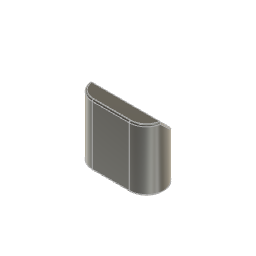
_Pencil Sharpener.d67306bd-12ad-4b4e-934f-6ecedd9aaf55 (Autodesk Fusion 360 design; units mm, degrees)
Autodesk Fusion 360 part; units mm, degrees
sketch "Sketch1" plane through (0, 0, 0) normal (0, 0, 1) x (1, 0, 0)
  circle A0 centre (0, 0) radius 6.985
  line L0 (-15.7585, 8.6989) -> (15.7585, -8.6989) construction
  line L1 (15.7585, 8.6989) -> (-15.7585, -8.6989) construction
  arc A1 (-9.364, 8.6989) -> (-9.364, -8.6989) centre (-9.3009, 0) ccw
  line L2 (0, 0) -> (0, 2.54)
  arc A2 (9.364, -8.6989) -> (9.364, 8.6989) centre (9.3009, 0) ccw
  line L3 (-9.364, -8.6989) -> (9.364, -8.6989)
  line L4 (9.364, 8.6989) -> (-9.364, 8.6989)
  dimension "d1" = 13.97
  constraint coincident A0.centre L2.start
  constraint coincident L0 A0.centre
  constraint coincident L1 A0.centre
  constraint vertical L2
  constraint symmetric A1.start L2 A2.end
  constraint symmetric A1.end L2 A2.start
  constraint symmetric A1 L2 A2
  measures "d1" diameter of A0
extrude "Extrude1" add sketch "Sketch1" along normal blind 38.1
ref_plane "WorkPlane1" through (0, 0, 19.05) normal (-1, 0, 0) x (0, 0, 1)
sketch "Sketch2" plane through (0, 0, 38.1) normal (0, 0, 1) x (-1, 0, 0)
  circle A0 centre (0, 0) radius 6.985
  line L0 (-9.364, -8.6989) -> (9.364, -8.6989)
  arc A1 (9.364, -8.6989) -> (9.364, 8.6989) centre (9.3009, 0) ccw
  line L1 (9.364, 8.6989) -> (-9.364, 8.6989)
  arc A2 (-9.364, 8.6989) -> (-9.364, -8.6989) centre (-9.3009, 0) ccw
sketch "Sketch3" plane through (0, 0, 0) normal (-1, 0, 0) x (0, -1, 0)
  line L0 (-6.985, 38.1) -> (6.985, 38.1)
  line L1 (-6.985, 0) -> (6.985, 0)
  line L2 (-6.985, 38.1) -> (6.985, 38.1)
  line L3 (6.985, 38.1) -> (6.985, 0)
  line L4 (6.985, 0) -> (-6.985, 0)
  line L5 (-6.985, 0) -> (-6.985, 38.1)
  line L6 (6.985, 38.1) -> (-6.985, 24.13)
  line L7 (6.985, 38.1) -> (26.7416, 38.1) construction
  line L8 (-6.985, 24.13) -> (-8.89, 24.13)
  line L9 (-8.89, 24.13) -> (-8.89, 38.1)
  line L10 (-8.89, 38.1) -> (-6.985, 38.1)
  line L11 (-6.985, 38.1) -> (-6.985, 24.13)
  line L12 (-6.985, 24.13) -> (0, 24.13)
  line L13 (0, 24.13) -> (0, 25.4)
  line L14 (0, 25.4) -> (-6.985, 25.4)
  line L15 (-6.985, 25.4) -> (-6.985, 24.13)
  line L16 (-6.985, 24.13) -> (-5.715, 25.4)
  line L17 (0, 25.4) -> (0, 31.115)
  line L18 (0, 31.115) -> (-6.985, 31.115)
  line L19 (6.985, 36.9017) -> (-6.985, 22.9317)
  line L20 (6.985, 36.9017) -> (26.7416, 36.9017) construction
  line L21 (-6.985, 22.9317) -> (-8.8388, 21.0779)
  line L22 (-8.8388, 21.0779) -> (-8.89, 24.13)
  line L23 (0, 31.115) -> (9.144, 31.115)
  line L24 (9.144, 31.115) -> (9.144, 38.354)
  line L25 (9.144, 38.354) -> (0, 38.354)
  line L26 (0, 38.354) -> (0, 31.115)
  dimension "d7" = 135
  dimension "d11" = 135
  constraint horizontal L2
  constraint vertical L3
  constraint horizontal L4
  constraint vertical L5
  constraint coincident L1.end L3.end
  constraint coincident L0.start L2.start
  constraint horizontal L7
  constraint coincident L0.end L2.end
  constraint coincident L5 L6.end
  constraint horizontal L8
  constraint vertical L9
  constraint horizontal L10
  constraint vertical L11
  constraint horizontal L12
  constraint vertical L13
  constraint horizontal L14
  constraint vertical L15
  constraint coincident L6 L16.end
  constraint coincident L14 L16.end
  constraint midpoint L6 L17.end
  constraint perpendicular L14 L17
  constraint midpoint L11 L18.end
  constraint horizontal L20
  constraint coincident L3 L19.start
  constraint coincident L5 L19.end
  constraint parallel L19 L21
  constraint horizontal L23
  constraint vertical L24
  constraint horizontal L25
  constraint vertical L26
  measures "d7" angle of L6 L7
  measures "d11" angle of L19 L20
revolve "Revolve1" add sketch "Sketch3" angle 360 about axis through (0, 0, 24.13) along (0, 0, 1) contours L5 L6 L11 L14 L18 | L5 L6 L11 L14 L15 L16
extrude "Extrude2" cut sketch "Sketch3" along normal mid plane 101.6 contours L0 L2 L5 L11 L18 L26 | L5 L8 L9 L10 L11 L15 | L0 L2 L3 L23 L24 L25 L26 | L0 L2 L6 L26 | L5 L6 L11 L14 L18 | L3 L6 L19 L23 | L6 L14 L17 L19 | L17 L19 L23 | L5 L6 L11 L14 L15 L16 | L5 L8 L21 L22 | L3 L19 L23 | L6 L12 L14 L16 L19 | L5 L12 L19
fillet "Fillet1" radius 0.762 7 edges at (15.8828, 5.688, 24.2287) (15.0365, -6.5404, 31.115) (0, -8.6989, 31.115) (-15.0365, -6.5404, 31.115) (-15.8828, 5.688, 24.2287) (0, 8.6989, 21.2179) (-6.5123, 2.5259, 0) 1 faces at (-0.174, 8.1211, 0)
